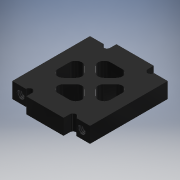
# Autodesk Inventor part: 上腕_メインフレーム_1_1
Saved by Autodesk Inventor 2018 (Build 220112000, 112)
## iProperties
Created: 2016-05-04
Part Number: 上腕_メインフレーム_1_1
Material: アセタール樹脂、黒
Document SubType Name: Modeling
Designer: hiroaki
Density: 1.425 g/cm^3
Appearance: 滑らか - 黒
Mass: 3.73288 g
Surface Area: 21.0392 cm^2
Volume: 2.61957 cm^3
d0: 25.000 mm
d1: 1.050 mm
d2: 2.000 mm
d3: 6.500 mm
d4: 3.100 mm
d6: 3.000 mm
d8: 3.000 mm
d9: 2.500 mm
d10: 2.500 mm
d11: 2.500 mm
d12: 2.500 mm
d13: 4.000 mm
d14: 2.500 mm
d15: 0.00 deg
d17: 5.000 mm
d18: 5.000 mm
d19: 2.700 mm
d21: 6.000 mm
d25: 8.800 mm
d27: 2.000 ul
d28: 360.00 deg
d30: 2.000 mm
Author: hiroaki
Autodesk Inventor part; units mm, degrees
ref_plane "YZ Plane" through (0, 0, 0) normal (1, 0, 0) x (0, 1, 0)
ref_plane "XZ Plane" through (0, 0, 0) normal (0, 1, 0) x (-1, 0, 0)
ref_plane "XY Plane" through (0, 0, 0) normal (0, 0, 1) x (1, 0, 0)
sketch "スケッチ1" plane through (0, 0, 0) normal (0, 0, 1) x (1, 0, 0)
  line L0 (-12.5, -12.5) -> (12.5, -12.5) construction
  line L1 (12.5, -12.5) -> (12.5, 12.5) construction
  line L2 (12.5, 12.5) -> (-12.5, 12.5) construction
  line L3 (-12.5, 12.5) -> (-12.5, -12.5) construction
  line L4 (-12.5, -12.5) -> (12.5, 12.5) construction
  line L5 (12.5, -12.5) -> (-12.5, 12.5) construction
  line L6 (-8.1, 12.5) -> (-12.5, 12.5)
  line L7 (-12.5, 12.5) -> (-12.5, 8.1)
  line L8 (8.1, 12.5) -> (12.5, 12.5)
  line L9 (12.5, 12.5) -> (12.5, 8.1)
  line L10 (-12.5, -8.1) -> (-12.5, -12.5)
  line L11 (-12.5, -12.5) -> (-8.1, -12.5)
  line L12 (8.1, -12.5) -> (12.5, -12.5)
  line L13 (12.5, -12.5) -> (12.5, -8.1)
  line L14 (-6, 12.5) -> (-6, 14.5)
  line L15 (-6, 14.5) -> (6, 14.5)
  line L16 (6, 14.5) -> (6, 12.5)
  arc A0 (-8.1, 12.5) -> (-6, 12.5) centre (-7.05, 12.5) ccw
  arc A1 (6, 12.5) -> (8.1, 12.5) centre (7.05, 12.5) ccw
  line L17 (0, 12.5) -> (0, 0) construction
  line L18 (0, 0) -> (12.5, 0) construction
  line L19 (-12.5, 6) -> (-14.5, 6) construction
  line L20 (-14.5, 6) -> (-14.5, -6) construction
  line L21 (-14.5, -6) -> (-12.5, -6) construction
  arc A2 (-12.5, 6) -> (-12.5, 8.1) centre (-12.5, 7.05) ccw
  arc A3 (-12.5, -8.1) -> (-12.5, -6) centre (-12.5, -7.05) ccw construction
  line L22 (-6, -12.5) -> (-6, -14.5)
  line L23 (-6, -14.5) -> (6, -14.5)
  line L24 (6, -14.5) -> (6, -12.5)
  arc A4 (-6, -12.5) -> (-8.1, -12.5) centre (-7.05, -12.5) ccw
  arc A5 (8.1, -12.5) -> (6, -12.5) centre (7.05, -12.5) ccw
  line L25 (12.5, 6) -> (14.5, 6) construction
  line L26 (14.5, 6) -> (14.5, -6) construction
  line L27 (14.5, -6) -> (12.5, -6) construction
  arc A6 (12.5, 8.1) -> (12.5, 6) centre (12.5, 7.05) ccw construction
  arc A7 (12.5, -6) -> (12.5, -8.1) centre (12.5, -7.05) ccw construction
  line L28 (-9.05, 12.5) -> (-5.95, 12.5) construction
  line L29 (-5.95, 12.5) -> (-5.95, 9.5) construction
  line L30 (-5.95, 9.5) -> (-9.05, 9.5) construction
  line L31 (-9.05, 9.5) -> (-9.05, 12.5) construction
  line L32 (-12.5, 9.05) -> (-9.5, 9.05) construction
  line L33 (-9.5, 9.05) -> (-9.5, 5.95) construction
  line L34 (-9.5, 5.95) -> (-12.5, 5.95) construction
  line L35 (-12.5, 5.95) -> (-12.5, 9.05) construction
  line L36 (-6.7322, 8.5) -> (6.7322, 8.5)
  line L37 (6.7322, 8.5) -> (0, 1.7678)
  line L38 (0, 1.7678) -> (-6.7322, 8.5)
  line L39 (-8.5, 6.7322) -> (-8.5, -6.7322)
  line L40 (-8.5, -6.7322) -> (-1.7678, 0)
  line L41 (-1.7678, 0) -> (-8.5, 6.7322)
  line L42 (-6.7322, -8.5) -> (6.7322, -8.5)
  line L43 (6.7322, -8.5) -> (0, -1.7678)
  line L44 (0, -1.7678) -> (-6.7322, -8.5)
  line L45 (8.5, 6.7322) -> (8.5, -6.7322)
  line L46 (8.5, -6.7322) -> (1.7678, 0)
  line L47 (1.7678, 0) -> (8.5, 6.7322)
  line L48 (-7.5, 12.5) -> (-7.5, 9.5) construction
  line L49 (-9.5, 7.5) -> (-12.5, 7.5) construction
  line L50 (-12.5, -12.5) -> (-12.5, 12.5)
  line L51 (12.5, -12.5) -> (12.5, 12.5)
  dimension "d0" = 25
  dimension "d1" = 1.05
  dimension "d2" = 2
  dimension "d3" = 6.5
  dimension "d4" = 3.1
  dimension "d6" = 3
  dimension "d8" = 3
  dimension "d9" = 2.5
  dimension "d10" = 2.5
  dimension "d11" = 2.5
  dimension "d12" = 2.5
  dimension "d13" = 4
  dimension "d17" = 5
  dimension "d18" = 5
  dimension "d31" = 25
  constraints: 104 end point, 16 perpendicular, 16 point on circle, 13 parallel, 9 horizontal, 8 centre point, 8 midpoint, 8 tangent, 7 equal radius, 6 collinear, 6 equal length, 6 symmetric about line, 5 vertical, 4 horizontal alignment, 4 vertical alignment, 10 other
  measures "d0" distance of L2.end L0.start
  measures "d1" radius of A0
  measures "d2" distance between parallel lines of L2 L15
  measures "d3" distance between parallel lines of L3 L14
  measures "d4" distance of L28.start L28.end
  measures "d6" distance between parallel lines of L6 L30
  measures "d8" distance between parallel lines of L3 L33
  measures "d9" distance between parallel lines of L43 L46
  measures "d10" distance between parallel lines of L41 L38
  measures "d11" distance between parallel lines of L47 L37
  measures "d12" distance between parallel lines of L44 L40
  measures "d13" distance between parallel lines of L36 L2
  measures "d17" distance between parallel lines of L2 L49
  measures "d18" distance between parallel lines of L7 L48
  measures "d31" distance of L1.end L2.end
extrude "押し出し1" add sketch "スケッチ1" along normal blind 2.5
mirror "ミラー1" about plane through (0, 0, 0) normal (0, 0, -1) of "押し出し1"
sketch "スケッチ2" plane through (-12.5, -12.5, 2.5) normal (0, -1, 0) x (1, 0, 0)
  line L0 (0, -5) -> (0, 0) projected
  line L1 (6.5, 0) -> (18.5, 0) construction
  line L2 (12.5, 0) -> (12.5, -5) construction
  point P0 (12.5, -2.5)
  point P1 (2.7, -2.5)
  point P2 (22.3, -2.5)
  point P3 (0, -2.5)
  dimension "d19" = 2.7
  constraints: 2 end point, 2 horizontal alignment, 2 midpoint, 1 symmetric about line, 1 vertical
  measures "d19" distance from line of L0 point (2.7, -2.5)
hole "穴1" at (-9.8, -12.5, 0) at (9.8, -12.5, 0) direction (0, 1, 0) diameter 2.459 depth 8.8 thread size "M3x0.5" class "6H" standard "ISO Metric profile"
pattern_circular "円形状パターン1" count 2 over 360 about axis through (0, 0, -10) along (0, 0, 1) of "穴1"
fillet "フィレット1" radius 2 12 edges at (8.5, 6.7322, 0) (8.5, -6.7322, 0) (6.7322, -8.5, 0) (0, 1.7678, 0) (-1.7678, 0, 0) (-6.7322, -8.5, 0) (-8.5, -6.7322, 0) (6.7322, 8.5, 0) (-8.5, 6.7322, 0) (-6.7322, 8.5, 0) (0, -1.7678, 0) (1.7678, 0, 0)
equation "\"d8\" = d6"
equation "\"d10\" = d9"
equation "\"d11\" = d10"
equation "\"d12\" = d11"
equation "\"d18\" = d17"
